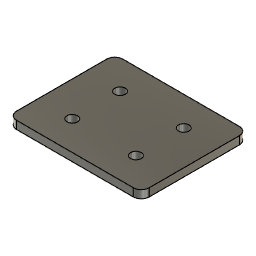
Platform_ gimbal (Autodesk Fusion 360 design; units mm, degrees)
Autodesk Fusion 360 part; units mm, degrees
sketch "Sketch1" plane through (0, 0, 0) normal (0, 0, 1) x (1, 0, 0)
  line L0 (0, 0) -> (-25, 0) construction
  line L1 (-25, 0) -> (-25, 17)
  line L2 (-22, 20) -> (0, 20)
  line L3 (0, 20) -> (0, 0) construction
  circle A0 centre (-12, 9) radius 2
  arc A1 (-22, 20) -> (-25, 17) centre (-22, 17) ccw
  circle A2 centre (-12, -9) radius 2
  arc A3 (-25, -17) -> (-22, -20) centre (-22, -17) ccw
  line L4 (-22, -20) -> (0, -20)
  line L5 (-25, 0) -> (-25, -17)
  arc A4 (25, 17) -> (22, 20) centre (22, 17) ccw
  arc A5 (22, -20) -> (25, -17) centre (22, -17) ccw
  line L6 (22, -20) -> (0, -20)
  line L7 (22, 20) -> (0, 20)
  line L8 (25, 0) -> (25, 17)
  circle A6 centre (12, -9) radius 2
  circle A7 centre (12, 9) radius 2
  line L9 (25, 0) -> (25, -17)
  point P0 (-25, 20)
  point P1 (-25, -20)
  point P2 (25, 20)
  point P3 (25, -20)
  dimension "d1" = 20
  dimension "d2" = 25
  dimension "d3" = 12
  dimension "d4" = 9
  dimension "d5" = 4
  dimension "d6" = 3
  constraint horizontal L0
  constraint vertical L1
  constraint horizontal L2
  constraint vertical L3
  constraint coincident L0.start L3.end
  constraint coincident P0 L1
  constraint coincident P0 L2
  constraint tangent L1 A1
  constraint tangent L2 A1
  constraint symmetric L3.end L0 origin
  constraint symmetric L1.start L0 L5.start
  constraint symmetric P0 L0 P1
  constraint symmetric L2.end L0 L4.end
  constraint symmetric L0 A0 A2
  constraint symmetric L0 L1.end A3.start
  constraint symmetric L0 L2.start A3.end
  constraint symmetric L0 A1 A3
  constraint symmetric L0.start L3 origin
  constraint symmetric L0.end L3 L8.start
  constraint symmetric P0 L3 P2
  constraint symmetric L2.end L3 L7.end
  constraint symmetric L3 A0 A7
  constraint symmetric L3 L1.end A4.start
  constraint symmetric L3 L2.start A4.end
  constraint symmetric L3 A1 A4
  constraint symmetric L3 L4.end L6.end
  constraint symmetric L3 L0.end L8.start
  constraint symmetric L3 L0.start origin
  constraint symmetric L3 A3.start A5.end
  constraint symmetric L3 A3.end A5.start
  constraint symmetric L3 P1 P3
  constraint symmetric L3 A2 A6
  constraint symmetric L3 A3 A5
  measures "d1" distance of L0.end P0
  measures "d2" distance of P0 L2.end
  measures "d3" distance of L3 A0.centre
  measures "d4" distance of L0 A0.centre
  measures "d5" diameter of A0
  measures "d6" radius of A1
extrude "Extrude1" add sketch "Sketch1" along normal blind 3
